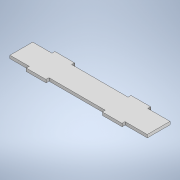
# Autodesk Inventor part: BungaSign-Bigger-Sides-LeftRight
Saved by Autodesk Inventor 2022 (Build 260153000, 153)
## iProperties
Created: 2022-08-22
Part Number: BungaSign-Bigger-Sides-LeftRight
Material: Generic
Document SubType Name: Modeling
Designer: incep
Density: 1 g/cm^3
Appearance: Default
Author: incep
Autodesk Inventor part; units mm, degrees
ref_plane "YZ Plane" through (0, 0, 0) normal (1, 0, 0) x (0, 1, 0)
ref_plane "XZ Plane" through (0, 0, 0) normal (0, 1, 0) x (-1, 0, 0)
ref_plane "XY Plane" through (0, 0, 0) normal (0, 0, 1) x (1, 0, 0)
sketch "Sketch1" plane through (0, 0, 0) normal (0, 1, 0) x (-1, 0, 0)
  line L0 (71, -11.5) -> (-71, -11.5)
  line L1 (-71, -11.5) -> (-71, 11.5)
  line L2 (-71, 11.5) -> (71, 11.5)
  line L3 (71, 11.5) -> (71, -11.5)
  line L4 (68, -11.5) -> (68, 11.5)
  line L5 (48.5, -14.5) -> (28.5, -14.5)
  line L6 (28.5, -14.5) -> (28.5, -11.5)
  line L7 (28.5, -11.5) -> (48.5, -11.5)
  line L8 (48.5, -11.5) -> (48.5, -14.5)
  line L9 (48.5, 11.5) -> (28.5, 11.5)
  line L10 (28.5, 11.5) -> (28.5, 14.5)
  line L11 (28.5, 14.5) -> (48.5, 14.5)
  line L12 (48.5, 14.5) -> (48.5, 11.5)
  line L13 (38.5, -14.5) -> (38.5, -11.5) construction
  line L14 (-48.5, -14.5) -> (-48.5, -11.5)
  line L15 (-38.5, -14.5) -> (-38.5, -11.5) construction
  line L16 (-48.5, -11.5) -> (-28.5, -11.5)
  line L17 (-28.5, 11.5) -> (-48.5, 11.5)
  line L18 (-28.5, -14.5) -> (-48.5, -14.5)
  line L19 (-48.5, 14.5) -> (-28.5, 14.5)
  line L20 (-28.5, 14.5) -> (-28.5, 11.5)
  line L21 (-28.5, -11.5) -> (-28.5, -14.5)
  line L22 (-48.5, 11.5) -> (-48.5, 14.5)
  point P0 (0, 0)
  point P1 (-71, 0)
  point P2 (0, -11.5)
  point P3 (48.5, -11.5)
  point P4 (28.5, -11.5)
  point P5 (-28.5, -11.5)
  point P6 (-48.5, -11.5)
  point P7 (-48.5, 11.5)
  point P8 (-28.5, 11.5)
  point P9 (28.5, 11.5)
  point P10 (48.5, 11.5)
  dimension "d0" = 23
  dimension "d1" = 142
  dimension "d2" = 3
  dimension "d3" = 20
  dimension "d4" = 3
  dimension "d5" = 20
  dimension "d6" = 3
  dimension "d7" = 38.5
  dimension "d10" = 77
  constraints: 46 end point, 6 parallel, 4 collinear, 4 horizontal, 4 midpoint, 4 perpendicular, 2 point on line, 1 horizontal alignment, 1 vertical alignment, 18 other
  measures "d0" distance of L0.end L1.end
  measures "d1" distance of L0.start L0.end
  measures "d2" distance between parallel lines of L4 L3
  measures "d3" distance of L5.start L5.end
  measures "d4" distance of L5.end L6.end
  measures "d5" distance of L10.end L11.end
  measures "d6" distance of L9.end L10.end
  measures "d7" distance from line of point (0, 0) L13
  measures "d10" distance of L6.end L14.end
extrude "Extrusion1" add sketch "Sketch1" along normal blind 3 contours L0 L1 L2 L4 | L8 L5 L6 L0 | L2 L10 L11 L12 | L21 L18 L14 L0 | L2 L22 L19 L20
equation "\"d0\" = stack"
equation "\"d3\" = finger"
equation "\"d4\" = thickness"
equation "\"d5\" = finger"
equation "\"d15\" = thickness"
equation "\"stack\" = 23"
equation "\"finger\" = 20"
equation "\"thickness\" = 3"
body "Solid1"
